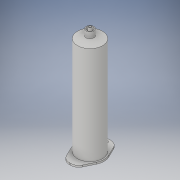
# Autodesk Inventor part: CH_01_0006_syringe
Saved by Autodesk Inventor 2019 (Build 230136000, 136)
## iProperties
Created: 2022-02-23
Part Number: CH_01_0006_syringe
Material: Generic
Document SubType Name: Modeling
Designer: Tomasz Krakowski
Density: 1 g/cm^3
Appearance: Default
Author: Tomasz Krakowski
Autodesk Inventor part; units mm, degrees
ref_plane "YZ Plane" through (0, 0, 0) normal (1, 0, 0) x (0, 1, 0)
ref_plane "XZ Plane" through (0, 0, 0) normal (0, 1, 0) x (-1, 0, 0)
ref_plane "XY Plane" through (0, 0, 0) normal (0, 0, 1) x (1, 0, 0)
sketch "Sketch1" plane through (0, 0, 0) normal (0, 1, 0) x (-1, 0, 0)
  circle A0 centre (0, 0) radius 14
  line L0 (0.7278, -24) -> (-0.7278, -24)
  line L1 (-0.7278, 24) -> (0.7278, 24)
  line L2 (16.75, 0) -> (0, 0) construction
  line L3 (0, 24) -> (0, 0) construction
  line L4 (0, 0) -> (0, -24) construction
  line L5 (-28.5847, 0) -> (0, 0) construction
  line L6 (9.7305, 18.3534) -> (15.0795, 7.2919)
  line L7 (9.7305, -18.3534) -> (15.0795, -7.2919)
  line L8 (-9.7305, 18.3534) -> (-15.0795, 7.2919)
  line L9 (-9.7305, -18.3534) -> (-15.0795, -7.2919)
  arc A1 (-15.0795, 7.2919) -> (-15.0795, -7.2919) centre (0, 0) ccw
  arc A2 (15.0795, -7.2919) -> (15.0795, 7.2919) centre (0, 0) ccw
  arc A3 (9.7305, 18.3534) -> (0.7278, 24) centre (0.7278, 14) ccw
  arc A4 (-0.7278, 24) -> (-9.7305, 18.3534) centre (-0.7278, 14) ccw
  arc A5 (0.7278, -24) -> (9.7305, -18.3534) centre (0.7278, -14) ccw
  arc A6 (-9.7305, -18.3534) -> (-0.7278, -24) centre (-0.7278, -14) ccw
  point P0 (-7, 24)
  point P1 (7, 24)
  dimension "d0" = 28
  dimension "d3" = 16.75
  dimension "d4" = 48
  dimension "d5" = 14
  dimension "d6" = 10
  constraints: 20 end point, 13 point on circle, 12 tangent, 7 centre point, 4 equal radius, 4 point on line, 2 coincident, 2 equal length, 2 horizontal, 2 midpoint, 2 vertical, 1 collinear, 1 parallel
  measures "d0" diameter of A0
  measures "d3" radius of A2
  measures "d4" distance between parallel lines of L0 L1
  measures "d5" distance of point (7, 24) point (-7, 24)
  measures "d6" radius of A3
extrude "Extrusion1" add sketch "Sketch1" along normal blind 2
sketch "Sketch2" plane through (0, 2, 0) normal (0, 1, 0) x (1, 0, 0)
  circle A0 centre (0, 0) radius 15
  circle A1 centre (0, 0) radius 14
  circle A2 centre (0, 0) radius 14 construction
  dimension "d9" = 30
  constraints: 2 centre point, 2 coincident, 1 concentric
  measures "d9" diameter of A0
extrude "Extrusion2" add sketch "Sketch2" along normal blind 117
sketch "Sketch5" plane through (0, 0, 0) normal (1, 0, 0) x (0, 1, 0)
  line L0 (0, 14) -> (119, 14) construction
  line L1 (118.2507, 14) -> (121.1776, 4)
  line L2 (2, 15) -> (119, 15) construction
  line L3 (119, 15) -> (122, 4.75)
  line L4 (0, 0) -> (118.2507, 0) construction
  line L5 (118.2507, 0) -> (118.2507, 14) construction
  line L6 (122, 4.75) -> (129, 4.75)
  line L7 (129, 4.75) -> (129, 3.75)
  line L8 (129, 3.75) -> (124, 3.75)
  line L9 (124, 3.75) -> (124, 1.75)
  line L10 (124, 1.75) -> (131.2, 1.75)
  line L11 (131.2, 1.75) -> (131.2, 1.25)
  line L12 (131.2, 1.25) -> (122.1776, 1.25)
  line L13 (121.1776, 4) -> (122.1776, 4)
  line L14 (122.1776, 4) -> (122.1776, 1.25)
  line L15 (119, 15) -> (119, 14)
  line L16 (119, 14) -> (118.2507, 14)
  dimension "d20" = 1
  dimension "d21" = 4.75
  dimension "d22" = 3
  dimension "d23" = 1
  dimension "d24" = 7
  dimension "d25" = 2.2
  dimension "d26" = 2
  dimension "d27" = 1.25
  dimension "d28" = 5
  dimension "d29" = 4
  dimension "d31" = 1
  constraints: 30 end point, 9 perpendicular, 4 horizontal, 1 parallel, 1 point on line
  measures "d20" distance between parallel lines of L3 L1
  measures "d21" distance from line of L4.end L6
  measures "d22" horizontal distance of L3.end L2.end
  measures "d23" distance between parallel lines of L6 L8
  measures "d24" distance from line of L7 L3.end
  measures "d25" distance between parallel lines of L11 L7
  measures "d26" distance between parallel lines of L10 L8
  measures "d27" distance between parallel lines of L4 L12
  measures "d28" distance between parallel lines of L7 L9
  measures "d29" distance between parallel lines of L4 L13
  measures "d31" distance from line of L14 L1.end
revolve "Revolution2" add sketch "Sketch5" angle 360 about axis through (0, 0, 0) along (0, 1, 0)
sketch "Sketch6" plane through (0, 0, 0) normal (0, -1, 0) x (1, 0, 0)
  circle A0 centre (0, -20) radius 1.75
  line L0 (0, -20) -> (0, 0) construction
  dimension "d33" = 3.5
  dimension "d34" = 20
  constraints: 2 end point, 1 centre point, 1 vertical
  measures "d33" diameter of A0
  measures "d34" distance of L0.end L0.start
extrude "Extrusion4" cut sketch "Sketch6" against normal up to surface (2 mm away)
body "Solid1"
